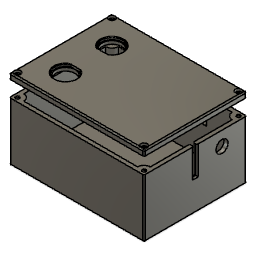
PCB-Box v8 (Autodesk Fusion 360 design; units mm, degrees)
Autodesk Fusion 360 part; units mm, degrees
note: some values were not read from the file. Set by a fixed rule: which sketch regions a step uses.
sketch "Sketch1" plane through (0, 0, 0) normal (0, 1, 0) x (1, 0, 0)
  circle A0 centre (-41.9037, 23.5706) radius 0.85
  circle A1 centre (22.0963, 23.5706) radius 0.85
  circle A2 centre (-41.9037, -20.4294) radius 0.85
  circle A3 centre (22.0963, -20.4294) radius 0.85
  circle A4 centre (-41.9037, 23.5706) radius 5
  circle A5 centre (22.0963, 23.5706) radius 5
  circle A6 centre (-41.9037, -20.4294) radius 5
  circle A7 centre (22.0963, -20.4294) radius 5
  line L0 (-51.9037, 33.5706) -> (32.0963, 33.5706)
  line L1 (32.0963, 33.5706) -> (32.0963, -30.4294)
  line L2 (32.0963, -30.4294) -> (-51.9037, -30.4294)
  line L3 (-51.9037, -30.4294) -> (-51.9037, 33.5706)
  line L4 (-51.9037, 33.5706) -> (-49.4037, 33.5706)
  line L5 (-49.4037, 33.5706) -> (-49.4037, -30.4294)
  line L6 (-49.4037, -30.4294) -> (-51.9037, -30.4294)
  line L7 (-51.9037, -30.4294) -> (-51.9037, 33.5706)
  line L8 (32.0963, 33.5706) -> (29.5963, 33.5706)
  line L9 (29.5963, 33.5706) -> (29.5963, -30.4294)
  line L10 (29.5963, -30.4294) -> (32.0963, -30.4294)
  line L11 (32.0963, -30.4294) -> (32.0963, 33.5706)
  line L12 (-49.4037, 33.5706) -> (29.5963, 33.5706)
  line L13 (29.5963, 33.5706) -> (29.5963, 31.0706)
  line L14 (29.5963, 31.0706) -> (-49.4037, 31.0706)
  line L15 (-49.4037, 31.0706) -> (-49.4037, 33.5706)
  line L16 (-49.4037, -30.4294) -> (29.5963, -30.4294)
  line L17 (29.5963, -30.4294) -> (29.5963, -27.9294)
  line L18 (29.5963, -27.9294) -> (-49.4037, -27.9294)
  line L19 (-49.4037, -27.9294) -> (-49.4037, -30.4294)
  point P0 (-41.9037, 23.5706)
  point P1 (22.0963, 23.5706)
  point P2 (-41.9037, -20.4294)
  point P3 (-41.9037, -20.4294)
  point P4 (22.0963, -20.4294)
  dimension "d8" = 64
  dimension "d12" = 44
  dimension "d13" = 64
  dimension "d14" = 44
  dimension "d16" = 1.7
  dimension "d17" = 1.7
  dimension "d18" = 1.7
  dimension "d19" = 1.7
  dimension "d21" = 10
  dimension "d22" = 10
  dimension "d23" = 10
  dimension "d24" = 10
  dimension "d28" = 84
  dimension "d29" = 64
  dimension "d30" = 10
  dimension "d31" = 10
  dimension "d32" = 10
  dimension "d33" = 10
  dimension "d34" = 2.5
  dimension "d35" = 64
  dimension "d36" = 2.5
  dimension "d37" = 64
  dimension "d38" = 79
  dimension "d39" = 2.5
  dimension "d40" = 79
  dimension "d41" = 2.5
  constraint coincident P2 A2.centre
  constraint coincident P0 A0.centre
  constraint coincident P1 A1.centre
  constraint coincident P3 P2
  constraint coincident P4 A3.centre
  constraint concentric A0 A4
  constraint concentric A1 A5
  constraint concentric A3 A7
  constraint horizontal L0
  constraint vertical L1
  constraint horizontal L2
  constraint vertical L3
  constraint horizontal L4
  constraint vertical L5
  constraint horizontal L6
  constraint vertical L7
  constraint horizontal L8
  constraint vertical L9
  constraint horizontal L10
  constraint vertical L11
  constraint horizontal L12
  constraint vertical L13
  constraint horizontal L14
  constraint vertical L15
  constraint horizontal L16
  constraint vertical L17
  constraint horizontal L18
  constraint vertical L19
  measures "d8" distance of P0 A1.centre
  measures "d12" distance of P0 P2
  measures "d13" distance of P3 A3.centre
  measures "d14" distance of P1 P4
  measures "d16" diameter of A0
  measures "d17" diameter of A1
  measures "d18" diameter of A2
  measures "d19" diameter of A3
  measures "d21" diameter of A4
  measures "d22" diameter of A5
  measures "d23" diameter of A6
  measures "d24" diameter of A7
  measures "d28" distance of L0.start L0.end
  measures "d29" distance of L0 L2
  measures "d30" distance of P0 L0
  measures "d31" distance of P1 L0
  measures "d32" distance of P0 L3
  measures "d33" distance of P2 L3
  measures "d34" distance of L0.start L4.end
  measures "d35" distance of L0.start L2.end
  measures "d36" distance of L0.end L8.end
  measures "d37" distance of L0.end L1.end
  measures "d38" distance of L4.end L8.end
  measures "d39" distance of L0 L14
  measures "d40" distance of L5.end L9.end
  measures "d41" distance of L5.end L18.end
extrude "Extrude1" add sketch "Sketch1" along normal blind 5 contours A4 | A5 | A6 | A7 makes body 1 at (27.0901, 3.3333, -23.3213) makes body 2 at (-36.9099, 3.3333, 20.6787) makes body 3 at (-36.9099, 3.3333, -23.3213) makes body 4 at (27.0901, 3.3333, 20.6787)
extrude "Extrude2" add sketch "Sketch1" along normal blind 34 separate body contours L0 L2 L3 L4 L5 L6 L7 L15 L19 | L0 L5 L9 L12 L13 L14 L15 | L0 L1 L2 L8 L9 L10 L11 L13 L17 | L2 L5 L9 L16 L17 L18 L19 makes body 5
extrude "Extrude3" add sketch "Sketch1" against normal blind 2.5 contours A0 | A1 | A2 | A3 | A4 | A5 | A6 | A7 | L0 L2 L3 L4 L5 L6 L7 L15 L19 | L0 L5 L9 L12 L13 L14 L15 | L0 L1 L2 L8 L9 L10 L11 L13 L17 | L5 L9 L14 L18 | L2 L5 L9 L16 L17 L18 L19 bodies 1 2 3 4 5
sketch "Sketch2" plane through (0, 34, 0) normal (0, 1, 0) x (-1, 0, 0)
  line L0 (49.4037, -31.0706) -> (-29.5963, -31.0706)
  line L1 (-29.5963, -31.0706) -> (-29.5963, 27.9294)
  line L2 (-29.5963, 27.9294) -> (49.4037, 27.9294)
  line L3 (49.4037, 27.9294) -> (49.4037, -31.0706)
  line L4 (51.9037, 30.4294) -> (-32.0963, 30.4294)
  line L5 (-32.0963, 30.4294) -> (-32.0963, -33.5706)
  line L6 (-32.0963, -33.5706) -> (51.9037, -33.5706)
  line L7 (51.9037, -33.5706) -> (51.9037, 30.4294)
  line L8 (-32.0963, 30.4294) -> (-32.0963, -33.5706)
  line L9 (-32.0963, 30.4294) -> (51.9037, 30.4294)
  line L10 (51.9037, 30.4294) -> (51.9037, -33.5706)
  line L11 (51.9037, -33.5706) -> (-32.0963, -33.5706)
  line L12 (-29.5963, -31.0706) -> (49.4037, -31.0706)
  line L13 (-29.5963, -33.5706) -> (-29.5963, 30.4294)
  line L14 (-29.5963, 27.9294) -> (49.4037, 27.9294)
  line L15 (49.4037, -33.5706) -> (49.4037, 30.4294)
  arc A0 (-29.5963, 23.9294) -> (-25.5963, 27.9294) centre (-29.5963, 27.9294) ccw
  arc A1 (-25.5963, -31.0706) -> (-29.5963, -27.0706) centre (-29.5963, -31.0706) ccw
  arc A2 (49.4037, -27.0706) -> (45.4037, -31.0706) centre (49.4037, -31.0706) ccw
  arc A3 (45.4037, 27.9294) -> (49.4037, 23.9294) centre (49.4037, 27.9294) ccw
  line L16 (-29.5963, 23.9294) -> (-29.5963, 27.9294)
  line L17 (-29.5963, -27.0706) -> (-29.5963, -31.0706)
  line L18 (45.4037, -31.0706) -> (49.4037, -31.0706)
  line L19 (45.4037, 27.9294) -> (49.4037, 27.9294)
  circle A4 centre (49.4037, 27.9294) radius 0.85
  circle A5 centre (-29.5963, 27.9294) radius 0.85
  circle A6 centre (-29.5963, -31.0706) radius 0.85
  circle A7 centre (49.4037, -31.0706) radius 0.85
  dimension "d48" = 4
  dimension "d49" = 4
  dimension "d50" = 4
  dimension "d51" = 4
  dimension "d54" = 1.7
  dimension "d55" = 1.7
  dimension "d56" = 1.7
  dimension "d57" = 1.7
  constraint coincident L1.end L2.start
  constraint coincident L0.end L1.start
  constraint coincident L0.start L3.end
  constraint coincident L14 A3.start
  constraint coincident L2.end L3.start
  constraint perpendicular L14 L16
  constraint perpendicular L12 L17
  constraint perpendicular L15 L18
  measures "d48" radius of A0
  measures "d49" radius of A1
  measures "d50" radius of A2
  measures "d51" radius of A3
  measures "d54" diameter of A4
  measures "d55" diameter of A5
  measures "d56" diameter of A6
  measures "d57" diameter of A7
extrude "Extrude4" add sketch "Sketch2" against normal blind 6 separate body contours L0 L3 L12 L15 A2 L18 A7 | L0 L3 L12 L15 L18 A7 makes body 6
extrude "Extrude5" add sketch "Sketch2" against normal blind 6 separate body contours L2 L3 L14 L15 A3 L19 A4 | L2 L3 L14 L15 L19 A4 makes body 7
extrude "Extrude6" add sketch "Sketch2" against normal blind 6 separate body contours L1 L2 L13 L14 A0 L16 A5 | L1 L2 L13 L14 L16 A5 makes body 8
extrude "Extrude7" add sketch "Sketch2" against normal blind 6 separate body contours L0 L1 L12 L13 A1 L17 A6 | L0 L1 L12 L13 L17 A6 makes body 9
combine "Combine1" operation add target body 1 tool bodies 6 7 8 9
extrude "Extrude8" cut sketch "Sketch2" against normal blind 15 contours L1 L13 L16 A5 | L1 L2 L13 L14 L16 A5 | L2 L13 L14 A5 bodies 1
extrude "Extrude9" cut sketch "Sketch2" against normal blind 15 contours L0 L12 L13 A6 | L0 L1 L12 L13 L17 A6 | L1 L13 L17 A6 bodies 1
extrude "Extrude10" cut sketch "Sketch2" against normal blind 15 contours L0 L3 L12 L15 L18 A7 | L0 L12 L15 L18 A7 | L3 L15 A7 bodies 1
extrude "Extrude11" cut sketch "Sketch2" against normal blind 15 contours L2 L3 L14 L15 L19 A4 | L3 L15 A4 | L2 L14 L15 L19 A4 bodies 1
ref_plane "WorkPlane1" through (-9.9037, 44, -1.5706) normal (0, 1, 0) x (0, 0, 1)
sketch "TopCover" plane through (-10.9037, 44, -2.5706) normal (0, 1, 0) x (1, 0, 0)
  line L0 (43, -33) -> (43, 31)
  line L1 (-41, -33) -> (43, -33)
  line L2 (40.5, -30.5) -> (-38.5, -30.5)
  line L3 (40.5, 28.5) -> (40.5, -30.5)
  line L4 (40.5, 28.5) -> (-38.5, 28.5)
  line L5 (43, 31) -> (-41, 31)
  line L6 (-41, 31) -> (-41, -33)
  line L7 (-38.5, -30.5) -> (-38.5, 28.5)
  circle A0 centre (40.5, -30.5) radius 1.05
  circle A1 centre (40.5, 28.5) radius 1.05
  circle A2 centre (-38.5, 28.5) radius 1.05
  circle A3 centre (-38.5, -30.5) radius 1.05
  line L8 (-41, -33) -> (43, -33)
  line L9 (43, -33) -> (43, 31)
  line L10 (43, 31) -> (-41, 31)
  line L11 (-41, 31) -> (-41, -33)
  dimension "d84" = 2.1
  dimension "d85" = 2.1
  dimension "d86" = 2.1
  dimension "d87" = 2.1
  constraint coincident L2.start L3.end
  constraint coincident L3.start L4.start
  constraint coincident L4.end L7.end
  constraint coincident L2.end L7.start
  constraint horizontal L8
  constraint vertical L9
  constraint horizontal L10
  constraint vertical L11
  constraint coincident L0.end L5.start
  constraint coincident L1.start L6.end
  measures "d84" diameter of A0
  measures "d85" diameter of A1
  measures "d86" diameter of A2
  measures "d87" diameter of A3
extrude "Extrude12" add sketch "TopCover" along normal blind 3.5 separate body contours L0 L1 L5 L6 L8 L9 L10 L11 | L2 L3 L4 L7 A0 A1 A2 A3 makes body 10
sketch "TopOfTopCover" plane through (0, 47.5, 0) normal (0, 1, 0) x (-1, 0, 0)
  circle A0 centre (49.4037, -31.0706) radius 1.05
  circle A1 centre (-29.5963, 27.9294) radius 1.05
  circle A2 centre (49.4037, 27.9294) radius 1.05
  circle A3 centre (-29.5963, -31.0706) radius 1.05
  line L0 (51.9037, -33.5706) -> (51.9037, 30.4294)
  line L1 (51.9037, 30.4294) -> (-32.0963, 30.4294)
  line L2 (-32.0963, 30.4294) -> (-32.0963, -33.5706)
  line L3 (-32.0963, -33.5706) -> (51.9037, -33.5706)
  line L4 (49.4037, 27.9294) -> (49.4037, -31.0706)
  line L5 (-29.5963, -31.0706) -> (49.4037, -31.0706)
  line L6 (-29.5963, 27.9294) -> (49.4037, 27.9294)
  line L7 (-29.5963, -31.0706) -> (-29.5963, 27.9294)
  circle A4 centre (-29.5963, 27.9294) radius 2
  circle A5 centre (-29.5963, -31.0706) radius 2
  circle A6 centre (49.4037, -31.0706) radius 2
  circle A7 centre (49.4037, 27.9294) radius 2
  circle A8 centre (34.4037, 12.9294) radius 6.05
  circle A9 centre (34.4037, 12.9294) radius 6.75
  line L8 (27.6537, 6.7794) -> (41.1537, 6.7794)
  line L9 (-32.0963, -1.5706) -> (51.9037, -1.5706)
  circle A10 centre (34.4037, -16.0706) radius 6.05
  circle A11 centre (34.4037, -16.0706) radius 6.75
  line L10 (27.6537, -9.9206) -> (41.1537, -9.9206)
  dimension "d91" = 4
  dimension "d92" = 4
  dimension "d93" = 4
  dimension "d94" = 4
  dimension "d161" = 12.1
  dimension "d162" = 15
  dimension "d163" = 15
  dimension "d164" = 13.5
  dimension "d165" = 8.25
  dimension "d166" = 13.5
  dimension "d167" = 6.15
  constraint coincident A1.centre L6.start
  constraint coincident A3.centre L5.start
  constraint coincident A0.centre L4.end
  constraint coincident A2.centre L4.start
  constraint concentric A8 A9
  constraint horizontal L8
  constraint midpoint L2 L9.start
  constraint midpoint L0 L9.end
  constraint symmetric A8 L9 A10
  constraint symmetric A9 L9 A11
  constraint symmetric L8.start L9 L10.start
  constraint symmetric L8.end L9 L10.end
  measures "d91" diameter of A4
  measures "d92" diameter of A5
  measures "d93" diameter of A6
  measures "d94" diameter of A7
  measures "d161" diameter of A8
  measures "d162" distance of L4 A8.centre
  measures "d163" distance of L6 A8.centre
  measures "d164" diameter of A9
  measures "d165" distance of L4 L8.end
  measures "d166" distance of L8.start L8.end
  measures "d167" distance of A8.centre L8
extrude "Extrude13" cut sketch "TopOfTopCover" against normal blind 1.5 contours A0 L4 L5 A6 | A0 L4 L5 A6 bodies 10
extrude "Extrude14" cut sketch "TopOfTopCover" against normal blind 1.5 contours A3 L5 L7 A5 | A3 L5 L7 A5 bodies 10
extrude "Extrude15" cut sketch "TopOfTopCover" against normal blind 1.5 contours A1 L6 L7 A4 | A1 L6 L7 A4 bodies 10
extrude "Extrude16" cut sketch "TopOfTopCover" against normal blind 1.5 contours A2 L4 L6 A7 | A2 L4 L6 A7 bodies 10
sketch "Sketch5" plane through (0, 34, 0) normal (0, 1, 0) x (-1, 0, 0)
  circle A0 centre (49.4037, 27.9294) radius 0.85
  circle A1 centre (49.4037, -31.0706) radius 0.85
  circle A2 centre (-29.5963, -31.0706) radius 0.85
  circle A3 centre (-29.5963, 27.9294) radius 0.85
  line L0 (45.4037, -31.0706) -> (-25.5963, -31.0706)
  arc A4 (-25.5963, -31.0706) -> (-29.5963, -27.0706) centre (-29.5963, -31.0706) ccw
  line L1 (-29.5963, -27.0706) -> (-29.5963, 23.9294)
  arc A5 (-29.5963, 23.9294) -> (-25.5963, 27.9294) centre (-29.5963, 27.9294) ccw
  line L2 (-25.5963, 27.9294) -> (45.4037, 27.9294)
  arc A6 (45.4037, 27.9294) -> (49.4037, 23.9294) centre (49.4037, 27.9294) ccw
  line L3 (49.4037, 23.9294) -> (49.4037, -27.0706)
  arc A7 (49.4037, -27.0706) -> (45.4037, -31.0706) centre (49.4037, -31.0706) ccw
  line L4 (51.9037, 30.4294) -> (-32.0963, 30.4294)
  line L5 (-32.0963, 30.4294) -> (-32.0963, -33.5706)
  line L6 (-32.0963, -33.5706) -> (51.9037, -33.5706)
  line L7 (51.9037, -33.5706) -> (51.9037, 30.4294)
  line L8 (51.9037, 30.4294) -> (-32.0963, 30.4294)
  line L9 (-32.0963, 30.4294) -> (-32.0963, -33.5706)
  line L10 (-32.0963, -33.5706) -> (51.9037, -33.5706)
  line L11 (51.9037, -33.5706) -> (51.9037, 30.4294)
  line L12 (-32.0963, -0.5706) -> (-29.5963, -0.5706)
  line L13 (-29.5963, -0.5706) -> (-29.5963, -2.5706)
  line L14 (-29.5963, -2.5706) -> (-32.0963, -2.5706)
  line L15 (-32.0963, -2.5706) -> (-32.0963, -0.5706)
  dimension "d105" = 2.5
  dimension "d106" = 2
  dimension "d107" = 31
  constraint horizontal L12
  constraint vertical L13
  constraint horizontal L14
  constraint vertical L15
  constraint coincident L9 L12.start
  measures "d105" distance of L12.start L12.end
  measures "d106" distance of L12.start L14.end
  measures "d107" distance of L8 L12
extrude "Extrude17" cut sketch "Sketch5" against normal blind 17 contours L1 L5 L9 L12 L13 L14 L15 bodies 1
sketch "powerPlugSketch" plane through (32.0963, 0, 0) normal (1, 0, 0) x (0, 0, -1)
  line L0 (2.5706, 34) -> (2.5706, 17)
  line L1 (2.5706, 17) -> (0.5706, 17)
  line L2 (0.5706, 17) -> (0.5706, 34)
  line L3 (0.5706, 34) -> (-30.4294, 34)
  line L4 (-30.4294, 34) -> (-30.4294, -2.5)
  line L5 (-30.4294, -2.5) -> (33.5706, -2.5)
  line L6 (33.5706, -2.5) -> (33.5706, 34)
  line L7 (33.5706, 34) -> (2.5706, 34)
  line L8 (-30.4294, -2.5) -> (-30.4294, 34)
  line L9 (33.5706, -2.5) -> (-30.4294, -2.5)
  line L10 (33.5706, -2.5) -> (33.5706, 34)
  line L11 (2.5706, 34) -> (33.5706, 34)
  line L12 (-30.4294, 34) -> (0.5706, 34)
  line L13 (2.5706, 34) -> (2.5706, 17)
  line L14 (0.5706, 17) -> (0.5706, 34)
  line L15 (2.5706, 17) -> (0.5706, 17)
  line L16 (27.0706, 34) -> (27.0706, 28)
  line L17 (31.0706, 19) -> (31.0706, 0)
  line L18 (31.0706, 0) -> (31.0706, 19)
  line L19 (31.0706, 19) -> (31.0706, 28)
  line L20 (31.0706, 28) -> (31.0706, 34)
  line L21 (31.0706, 34) -> (31.0706, 28)
  line L22 (31.0706, 28) -> (31.0706, 19)
  circle A0 centre (18.2706, 25.2) radius 3.8
  dimension "d115" = 7.6
  dimension "d116" = 8.8
  dimension "d117" = 12.8
  measures "d115" diameter of A0
  measures "d116" distance of L7 A0.centre
  measures "d117" distance of L22 A0.centre
extrude "Extrude18" cut sketch "powerPlugSketch" against normal blind 2.5 contours A0 bodies 1
sketch "Sketch7" plane through (0, 0, -33.5706) normal (0, 0, -1) x (-1, 0, 0)
  line L0 (51.9037, -2.5) -> (51.9037, 34)
  line L1 (51.9037, 34) -> (-32.0963, 34)
  line L2 (-32.0963, 34) -> (-32.0963, -2.5)
  line L3 (-32.0963, -2.5) -> (51.9037, -2.5)
  line L4 (51.9037, -2.5) -> (51.9037, 34)
  line L5 (51.9037, -2.5) -> (-32.0963, -2.5)
  line L6 (-32.0963, 34) -> (51.9037, 34)
  line L7 (-32.0963, -2.5) -> (-32.0963, 34)
  line L8 (-9.5963, 34) -> (-0.5963, 34)
  line L9 (-0.5963, 34) -> (-0.5963, 18.5)
  line L10 (-0.5963, 18.5) -> (-9.5963, 18.5)
  line L11 (-9.5963, 18.5) -> (-9.5963, 34)
  dimension "d120" = 9
  dimension "d121" = 15.5
  dimension "d122" = 22.5
  constraint horizontal L8
  constraint vertical L9
  constraint horizontal L10
  constraint vertical L11
  constraint coincident L6 L8.start
  measures "d120" distance of L8.start L8.end
  measures "d121" distance of L8.start L10.end
  measures "d122" distance of L7 L11
extrude "Extrude19" cut sketch "Sketch7" against normal blind 2.5 contours L1 L6 L8 L9 L10 L11 bodies 1
fillet "Fillet1" radius 0.8 1 edges at (32.0963, 15.75, -33.5706) on bodies 1
fillet "Fillet2" radius 0.8 1 edges at (-51.9037, 15.75, -33.5706) on bodies 1
fillet "Fillet3" radius 0.8 1 edges at (32.0963, 15.75, 30.4294) on bodies 1
fillet "Fillet4" radius 0.8 1 edges at (-51.9037, 15.75, 30.4294) on bodies 1
fillet "Fillet5" radius 0.8 3 edges at (32.0963, 25.5, -2.5706) (32.0963, 17, -1.5706) (32.0963, 25.5, -0.5706) on bodies 1
fillet "Fillet6" radius 0.8 3 edges at (29.5963, 25.5, -0.5706) (29.5963, 17, -1.5706) (29.5963, 25.5, -2.5706) on bodies 1
fillet "Fillet7" radius 0.34 1 edges at (-48.6112, 34, 28.2368) on bodies 1
fillet "Fillet8" radius 0.34 1 edges at (30.3888, 34, 28.2368) on bodies 1
fillet "Fillet9" radius 0.34 1 edges at (30.3888, 34, -30.7632) on bodies 1
fillet "Fillet10" radius 0.34 1 edges at (-48.6112, 34, -30.7632) on bodies 1
fillet "Fillet11" radius 0.2833 1 edges at (-42.6962, 5, -23.8779) on bodies 1 3
fillet "Fillet12" radius 0.2833 1 edges at (21.3038, 5, -23.8779) on bodies 1
fillet "Fillet13" radius 0.2833 1 edges at (21.3038, 5, 20.1221) on bodies 1 4
fillet "Fillet14" radius 0.2833 1 edges at (-42.6962, 5, 20.1221) on bodies 1 2
fillet "Fillet15" radius 0.8 8 edges at (31.862, -2.5, -33.3363) (32.0963, -2.5, -1.5706) (31.862, -2.5, 30.1951) (-9.9037, -2.5, 30.4294) (-51.6694, -2.5, 30.1951) (-51.9037, -2.5, -1.5706) (-51.6694, -2.5, -33.3363) (-9.9037, -2.5, -33.5706) on bodies 1
fillet "Fillet16" radius 0.8 8 edges at (-9.9037, 47.5, -33.5706) (-51.9037, 47.5, -1.5706) (-9.9037, 47.5, 30.4294) (32.0963, 47.5, -1.5706) (32.0963, 45.75, -33.5706) (-51.9037, 45.75, -33.5706) (-51.9037, 45.75, 30.4294) (32.0963, 45.75, 30.4294) on bodies 10
extrude "Extrude20" cut sketch "TopOfTopCover" against normal blind 3.5 contours A8 bodies 10
extrude "Extrude21" cut sketch "TopOfTopCover" against normal blind 1.5 contours A9 L8 picked at (31.2488, 7.2419) bodies 10
extrude "Extrude22" cut sketch "TopOfTopCover" against normal blind 3.5 contours A10 bodies 10
extrude "Extrude23" cut sketch "TopOfTopCover" against normal blind 1.5 contours A11 L10 picked at (31.2488, -10.3831) bodies 10
fillet "Fillet17" radius 0.4 2 edges at (-34.4037, 47.5, -22.8206) (-34.4037, 47.5, 19.6794) on bodies 10
equation "HorizHoleSpacing = 64 mm"
equation "VertHoleSpacing = 44 mm"
equation "BoardBesideHole = 3.5 mm"
equation "BufferAroundBoard = 4 mm"
equation "PostHeight = 5 mm" comment "6mm screw, 1mm of which is taken up by board, and likely 1mm by the box"
equation "BoxWallWidth = 2.5 mm"
equation "HoleDepth = PostHeight + 1 mm"
equation "d8 = HorizHoleSpacing"
equation "d12 = VertHoleSpacing"
equation "d13 = HorizHoleSpacing"
equation "d14 = VertHoleSpacing"
equation "holeDia = 1.7 mm" comment "M2 outderDia=1.93, inner dia = 1.81"
equation "d16 = holeDia"
equation "d17 = holeDia"
equation "d18 = holeDia"
equation "d19 = holeDia"
equation "postDia = 10 mm"
equation "d21 = postDia"
equation "d22 = postDia"
equation "d23 = postDia"
equation "d24 = postDia"
equation "BoxLength = HorizHoleSpacing + 2 * ( BoardBesideHole + BufferAroundBoard + BoxWallWidth )"
equation "BoxWidth = VertHoleSpacing + 2 * ( BoardBesideHole + BufferAroundBoard + BoxWallWidth )"
equation "WallHeight = 29 mm + PostHeight"
equation "d28 = BoxLength"
equation "d29 = BoxWidth"
equation "d30 = BufferAroundBoard + BoardBesideHole + BoxWallWidth"
equation "d31 = BufferAroundBoard + BoardBesideHole + BoxWallWidth"
equation "d32 = BufferAroundBoard + BoardBesideHole + BoxWallWidth"
equation "d33 = BufferAroundBoard + BoardBesideHole + BoxWallWidth"
equation "d34 = BoxWallWidth"
equation "d35 = BoxWidth"
equation "d36 = BoxWallWidth"
equation "d37 = BoxWidth"
equation "d38 = BoxLength - ( 2 * BoxWallWidth )"
equation "d39 = BoxWallWidth"
equation "d40 = BoxLength - ( 2 * BoxWallWidth )"
equation "d41 = BoxWallWidth"
equation "d42 = PostHeight"
equation "d44 = WallHeight"
equation "d46 = -BoxWallWidth"
equation "d48 = BufferAroundBoard"
equation "d49 = BufferAroundBoard"
equation "d50 = BufferAroundBoard"
equation "d51 = BufferAroundBoard"
equation "TopScrewPostDepth = 6 mm"
equation "TopScrewHoleDepth = 15 mm"
equation "d54 = holeDia"
equation "d55 = holeDia"
equation "d56 = holeDia"
equation "d57 = holeDia"
equation "d58 = -TopScrewPostDepth"
equation "d60 = -TopScrewPostDepth"
equation "d62 = -TopScrewPostDepth"
equation "d64 = -TopScrewPostDepth"
equation "d66 = -TopScrewHoleDepth"
equation "d68 = -TopScrewHoleDepth"
equation "d70 = -TopScrewHoleDepth"
equation "d72 = -TopScrewHoleDepth"
equation "TopCoverExtraThickness = 3.5 mm"
equation "TopCoverInsetDepth = 2 mm"
equation "TopCoverInsetRimThickness = 3 mm"
equation "TopHoleDia = 2.1 mm"
equation "LidTolerance = 0.3 mm"
equation "TopCounterSinkDepth = 1.5 mm"
equation "TopCounterSinkDiameter = 4 mm"
equation "d84 = TopHoleDia"
equation "d85 = TopHoleDia"
equation "d86 = TopHoleDia"
equation "d87 = TopHoleDia"
equation "d88 = TopCoverExtraThickness"
equation "filletRadius = 0.8 mm"
equation "d91 = TopCounterSinkDiameter"
equation "d92 = TopCounterSinkDiameter"
equation "d93 = TopCounterSinkDiameter"
equation "d94 = TopCounterSinkDiameter"
equation "d95 = -TopCounterSinkDepth"
equation "d97 = -TopCounterSinkDepth"
equation "d99 = -TopCounterSinkDepth"
equation "d101 = -TopCounterSinkDepth"
equation "SlotWidth = 2 mm"
equation "SlotDepth = ( WallHeight / 2 )"
equation "d105 = BoxWallWidth"
equation "d106 = SlotWidth"
equation "d107 = ( BoxWidth / 2 ) - ( SlotWidth / 2 )"
equation "d108 = -SlotDepth"
equation "PowerPlugFromTop = 5 mm" comment "from top of hole to top of wall"
equation "PowerSwitchSlotWidth = 9 mm"
equation "PowerSwitchSlotDepth = 15.5 mm"
equation "PowerSwitchSlotFromEnd = 16 mm + BufferAroundBoard + BoxWallWidth"
equation "PowerPlugHoleDia = 7.6 mm"
equation "d115 = PowerPlugHoleDia"
equation "d116 = PowerPlugFromTop + ( PowerPlugHoleDia / 2 )"
equation "d117 = BufferAroundBoard + PowerPlugFromTop + ( PowerPlugHoleDia / 2 )"
equation "d118 = -BoxWallWidth"
equation "d120 = PowerSwitchSlotWidth"
equation "d121 = PowerSwitchSlotDepth"
equation "d122 = PowerSwitchSlotFromEnd"
equation "d123 = -BoxWallWidth"
equation "d126 = filletRadius"
equation "d128 = filletRadius"
equation "d130 = filletRadius"
equation "d132 = filletRadius"
equation "d134 = filletRadius"
equation "d136 = filletRadius"
equation "d138 = holeDia / 5"
equation "d140 = holeDia / 5"
equation "d142 = holeDia / 5"
equation "d144 = holeDia / 5"
equation "d146 = holeDia / 6"
equation "d148 = holeDia / 6"
equation "d150 = holeDia / 6"
equation "d152 = holeDia / 6"
equation "d154 = filletRadius"
equation "d156 = filletRadius"
equation "ButtonHoleDia = 13.5 mm"
equation "ButtonShortCut = ( ButtonHoleDia / 2 ) - ( ButtonHoleDia - 12.9 mm )"
equation "ButtonInnerHoleDia = 12.1 mm"
equation "ButtonFromSide = 15 mm"
equation "d161 = ButtonInnerHoleDia"
equation "d162 = ButtonFromSide"
equation "d163 = ButtonFromSide"
equation "d164 = ButtonHoleDia"
equation "d165 = ButtonFromSide - ( 0.5 * ButtonHoleDia )"
equation "d166 = ButtonHoleDia"
equation "d167 = ButtonShortCut"
equation "ButtonInsetDepth = 1.5 mm"
equation "d169 = -TopCoverExtraThickness"
equation "d171 = -ButtonInsetDepth"
equation "d173 = -TopCoverExtraThickness"
equation "d175 = -ButtonInsetDepth"
equation "d178 = filletRadius / 2"
named bodies: "MainBody", "TopCover"
